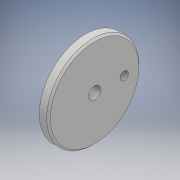
# Autodesk Inventor part: шайба концевая 50
Saved by Autodesk Inventor 2018.3 (Build 223284000, 284)
## iProperties
Created: 2018-05-21
Part Number: шайба концевая 50
Material: Типовые
Document SubType Name: Modeling
Designer: kriku
Density: 1 g/cm^3
Appearance: По умолчанию
Mass: 9.4894 g
Surface Area: 46.932 cm^2
Volume: 9.4894 cm^3
Author: kriku
Autodesk Inventor part; units mm, degrees
ref_plane "YZ Plane" through (0, 0, 0) normal (1, 0, 0) x (0, 1, 0)
ref_plane "XZ Plane" through (0, 0, 0) normal (0, 1, 0) x (-1, 0, 0)
ref_plane "XY Plane" through (0, 0, 0) normal (0, 0, 1) x (1, 0, 0)
sketch "Эскиз1" plane through (0, 0, 0) normal (1, 0, 0) x (0, 1, 0)
  circle A0 centre (0, 0) radius 25
  circle A1 centre (0, 0) radius 3.3
  circle A2 centre (16, 0) radius 2.25
  line L0 (-35, 0) -> (35, 0) projected
  dimension "d0" = 50
  dimension "d1" = 6.6
  dimension "d2" = 4.5
  dimension "d3" = 16
  constraints: 3 centre point, 2 coincident, 1 point on line
  measures "d0" diameter of A0
  measures "d1" diameter of A1
  measures "d2" diameter of A2
  measures "d3" distance of point (0, 0) A2.centre
extrude "Выдавливание1" add sketch "Эскиз1" along normal blind 5 contours L0 A2 A1 A0 | A0 L0 A1 A2
chamfer "Фаска1" distance 1 angle 45 1 edges at (5, -25, 0)
